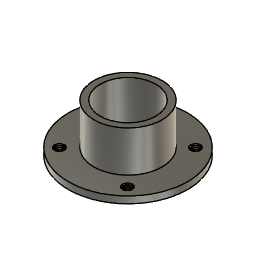
20mm_swivel (Autodesk Fusion 360 design; units mm, degrees)
Autodesk Fusion 360 part; units mm, degrees
sketch "Sketch1" plane through (0, 0, 0) normal (0, 0, 1) x (1, 0, 0)
  circle A0 centre (0, 0) radius 17.5
  dimension "d1" = 35
  constraint coincident A0.centre origin
  measures "d1" diameter of A0
extrude "Extrude1" add sketch "Sketch1" along normal blind 2
sketch "Sketch2" plane through (0, 0, 2) normal (0, 0, 1) x (-1, 0, 0)
  circle A0 centre (0, 0) radius 17.5
  line L0 (10, 10) -> (-10, 10) construction
  line L1 (-10, 10) -> (-10, -10) construction
  line L2 (-10, -10) -> (10, -10) construction
  line L3 (10, -10) -> (10, 10) construction
  circle A1 centre (10, -10) radius 1.5
  circle A2 centre (-10, -10) radius 1.5
  circle A3 centre (10, 10) radius 1.5
  circle A4 centre (-10, 10) radius 1.5
  dimension "d4" = 20
  dimension "d5" = 20
  dimension "d6" = 10
  dimension "d7" = 10
  dimension "d8" = 3
  dimension "d9" = 3
  dimension "d10" = 3
  dimension "d11" = 3
  constraint horizontal L0
  constraint vertical L1
  constraint horizontal L2
  constraint vertical L3
  constraint coincident L2.end L3.start
  constraint coincident L1.end L2.start
  constraint coincident L0.start L3.end
  constraint coincident L0.end L1.start
  measures "d4" distance of L0.start L0.end
  measures "d5" distance of L0.end L1.end
  measures "d6" distance of A0.centre L1
  measures "d7" distance of A0.centre L0
  measures "d8" diameter of A1
  measures "d9" diameter of A2
  measures "d10" diameter of A3
  measures "d11" diameter of A4
hole "Hole1" at (-10, 10, 2) at (10, 10, 2) at (10, -10, 2) at (-10, -10, 2) direction (0, 0, -1) diameter 2.529 depth 2 tip angle 118
thread "Thread1" "ISO Metric profile 3.0 M3x0.5 M3x0.5 6H" major diameter 3.086 minor diameter 2.529 pitch 0.5 angle 60 modelled right hand crest width 0.1368 on face at (-9.8741, -11.2582, 1.3333) crest through (-8.7355, -10, 1.875) on face at (10.1259, 8.7418, 1.3333) crest through (11.2645, 10, 1.875) on face at (10.1259, -11.2582, 1.3333) crest through (11.2645, -10, 1.875) on face at (-9.8741, 8.7418, 1.3333) crest through (-8.7355, 10, 1.875)
sketch "Sketch3" plane through (0, 0, 2) normal (0, 0, 1) x (-1, 0, 0)
  spline S0 degree 3 poles (-10.9581, 9.1748) (-11.0802, 9.2888) (-11.1784, 9.426) (-11.3207, 9.736) (-11.3611, 9.907) (-11.3757, 10.2618) (-11.3471, 10.4423) (-11.2212, 10.7891) (-11.1226, 10.9512) (-10.9156, 11.1792) (-10.8244, 11.2577) (-10.6232, 11.3929) (-10.5136, 11.4486) (-10.3985, 11.4906) knots 0 0 0 0 0.050111 0.050111 0.102261 0.102261 0.15645 0.15645 0.212677 0.212677 0.24852 0.24852 0.285143 0.285143 0.285143 0.285143
  arc A0 (-9.6015, 11.4906) -> (-10.3985, 11.4906) centre (-10, 10) ccw
  spline S1 degree 3 poles (-9.6015, 11.4906) (-9.4166, 11.4231) (-9.2465, 11.3207) (-8.9611, 11.0601) (-8.8468, 10.9065) (-8.6876, 10.5696) (-8.6419, 10.3908) (-8.6233, 10.0326) (-8.648, 9.8568) (-8.741, 9.5918) (-8.7875, 9.4972) (-8.901, 9.3235) (-8.967, 9.2447) (-9.0419, 9.1748) knots 0 0 0 0 0.059039 0.059039 0.116033 0.116033 0.170983 0.170983 0.223888 0.223888 0.255505 0.255505 0.286347 0.286347 0.286347 0.286347
  arc A1 (-10.9581, 9.1748) -> (-9.0419, 9.1748) centre (-10, 10) ccw
  spline S2 degree 3 poles (9.0419, -10.8252) (8.9198, -10.7112) (8.8216, -10.574) (8.6793, -10.264) (8.6389, -10.093) (8.6243, -9.7382) (8.6529, -9.5577) (8.7788, -9.2109) (8.8774, -9.0488) (9.0844, -8.8208) (9.1756, -8.7423) (9.3768, -8.6071) (9.4864, -8.5514) (9.6015, -8.5094) knots 0 0 0 0 0.050111 0.050111 0.102261 0.102261 0.15645 0.15645 0.212677 0.212677 0.24852 0.24852 0.285143 0.285143 0.285143 0.285143
  arc A2 (10.3985, -8.5094) -> (9.6015, -8.5094) centre (10, -10) ccw
  spline S3 degree 3 poles (10.3985, -8.5094) (10.5834, -8.5769) (10.7535, -8.6793) (11.0389, -8.9399) (11.1532, -9.0935) (11.3124, -9.4304) (11.3581, -9.6092) (11.3767, -9.9674) (11.352, -10.1432) (11.259, -10.4082) (11.2125, -10.5028) (11.099, -10.6765) (11.033, -10.7553) (10.9581, -10.8252) knots 0 0 0 0 0.059039 0.059039 0.116033 0.116033 0.170983 0.170983 0.223888 0.223888 0.255505 0.255505 0.286347 0.286347 0.286347 0.286347
  arc A3 (9.0419, -10.8252) -> (10.9581, -10.8252) centre (10, -10) ccw
  spline S4 degree 3 poles (-10.9581, -10.8252) (-11.0802, -10.7112) (-11.1784, -10.574) (-11.3207, -10.264) (-11.3611, -10.093) (-11.3757, -9.7382) (-11.3471, -9.5577) (-11.2212, -9.2109) (-11.1226, -9.0488) (-10.9156, -8.8208) (-10.8244, -8.7423) (-10.6232, -8.6071) (-10.5136, -8.5514) (-10.3985, -8.5094) knots 0 0 0 0 0.050111 0.050111 0.102261 0.102261 0.15645 0.15645 0.212677 0.212677 0.24852 0.24852 0.285143 0.285143 0.285143 0.285143
  arc A4 (-9.6015, -8.5094) -> (-10.3985, -8.5094) centre (-10, -10) ccw
  spline S5 degree 3 poles (-9.6015, -8.5094) (-9.4166, -8.5769) (-9.2465, -8.6793) (-8.9611, -8.9399) (-8.8468, -9.0935) (-8.6876, -9.4304) (-8.6419, -9.6092) (-8.6233, -9.9674) (-8.648, -10.1432) (-8.741, -10.4082) (-8.7875, -10.5028) (-8.901, -10.6765) (-8.967, -10.7553) (-9.0419, -10.8252) knots 0 0 0 0 0.059039 0.059039 0.116033 0.116033 0.170983 0.170983 0.223888 0.223888 0.255505 0.255505 0.286347 0.286347 0.286347 0.286347
  arc A5 (-10.9581, -10.8252) -> (-9.0419, -10.8252) centre (-10, -10) ccw
  spline S6 degree 3 poles (9.0419, 9.1748) (8.9198, 9.2888) (8.8216, 9.426) (8.6793, 9.736) (8.6389, 9.907) (8.6243, 10.2618) (8.6529, 10.4423) (8.7788, 10.7891) (8.8774, 10.9512) (9.0844, 11.1792) (9.1756, 11.2577) (9.3768, 11.3929) (9.4864, 11.4486) (9.6015, 11.4906) knots 0 0 0 0 0.050111 0.050111 0.102261 0.102261 0.15645 0.15645 0.212677 0.212677 0.24852 0.24852 0.285143 0.285143 0.285143 0.285143
  arc A6 (10.3985, 11.4906) -> (9.6015, 11.4906) centre (10, 10) ccw
  spline S7 degree 3 poles (10.3985, 11.4906) (10.5834, 11.4231) (10.7535, 11.3207) (11.0389, 11.0601) (11.1532, 10.9065) (11.3124, 10.5696) (11.3581, 10.3908) (11.3767, 10.0326) (11.352, 9.8568) (11.259, 9.5918) (11.2125, 9.4972) (11.099, 9.3235) (11.033, 9.2447) (10.9581, 9.1748) knots 0 0 0 0 0.059039 0.059039 0.116033 0.116033 0.170983 0.170983 0.223888 0.223888 0.255505 0.255505 0.286347 0.286347 0.286347 0.286347
  arc A7 (9.0419, 9.1748) -> (10.9581, 9.1748) centre (10, 10) ccw
  circle A8 centre (0, 0) radius 17.5
  circle A9 centre (0, 0) radius 10
  dimension "d17" = 20
  constraint concentric A8 A9
  measures "d17" diameter of A9
extrude "Extrude2" add sketch "Sketch3" along normal blind 12 contours A9
sketch "Sketch4" plane through (0, 0, 14) normal (0, 0, 1) x (-1, 0, 0)
  circle A0 centre (0, 0) radius 10
  circle A1 centre (0, 0) radius 8.15
  dimension "d20" = 16.3
  constraint coincident A0.centre A1.centre
  measures "d20" diameter of A1
extrude "Extrude3" cut sketch "Sketch4" against normal blind 15 contours A1
